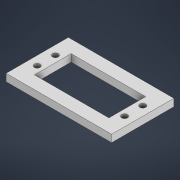
# Autodesk Inventor part: Servohalterung_v2
Saved by Autodesk Inventor 2021 (Build 250183000, 183)
## iProperties
Created: 2021-01-09
Part Number: Servohalterung_v2
Material: Generisch
Document SubType Name: Modeling
Designer: laure
Density: 1 g/cm^3
Appearance: Vorgabe
Author: laure
Autodesk Inventor part; units mm, degrees
ref_plane "YZ Plane" through (0, 0, 0) normal (1, 0, 0) x (0, 1, 0)
ref_plane "XZ Plane" through (0, 0, 0) normal (0, 1, 0) x (-1, 0, 0)
ref_plane "XY Plane" through (0, 0, 0) normal (0, 0, 1) x (1, 0, 0)
sketch "Skizze1" plane through (0, 0, 0) normal (0, 1, 0) x (-1, 0, 0)
  line L0 (20.5, -10.1) -> (-20.5, -10.1)
  line L1 (-20.5, -10.1) -> (-20.5, 10.1)
  line L2 (-20.5, 10.1) -> (20.5, 10.1)
  line L3 (20.5, 10.1) -> (20.5, -10.1)
  line L4 (0, -23.94) -> (0, 23.94) projected
  line L5 (-40.6, 0) -> (40.6, 0) projected
  line L6 (29, -17.1) -> (-29, -17.1)
  line L7 (-29, -17.1) -> (-29, 17.1)
  line L8 (-29, 17.1) -> (29, 17.1)
  line L9 (29, 17.1) -> (29, -17.1)
  point P0 (0, 0)
  dimension "d0" = 41
  dimension "d3" = 20.2
  dimension "d7" = 58
  dimension "d8" = 7
  constraints: 16 end point, 4 parallel, 2 horizontal, 2 perpendicular, 4 other
  measures "d0" distance between parallel lines of L1 L3
  measures "d3" distance of L2.end L0.start
  measures "d7" distance between parallel lines of L7 L9
  measures "d8" distance between parallel lines of L6 L0
extrude "Extrusion2" add sketch "Skizze1" along normal mid plane 4 contours L3 L5 L9 L6 L4 L0 | L4 L6 L7 L5 L1 L0 | L3 L2 L4 L8 L9 L5 | L5 L7 L8 L4 L2 L1
sketch "Skizze2" plane through (0, 2, 0) normal (0, 1, 0) x (1, 0, 0)
  circle A0 centre (-24, 5) radius 1.6
  circle A1 centre (-24, -5) radius 1.6
  line L0 (-29, 17.1) -> (-29, -17.1) projected
  line L1 (40.6, 0) -> (-40.6, 0) projected
  line L2 (0, 23.94) -> (0, -23.94) projected
  circle A2 centre (24, 5) radius 1.6
  circle A3 centre (24, -5) radius 1.6
  point P0 (0, 0)
  dimension "d11" = 3.2
  dimension "d12" = 3.2
  dimension "d13" = 5
  dimension "d14" = 5
  dimension "d15" = 10
  dimension "d16" = 5
  constraints: 4 centre point, 2 symmetric about line, 2 other
  measures "d11" diameter of A0
  measures "d12" diameter of A1
  measures "d13" distance from line of L0 A0.centre
  measures "d14" distance from line of L0 A1.centre
  measures "d15" distance of A1.centre A0.centre
  measures "d16" distance from line of L1 A0.centre
extrude "Extrusion3" cut sketch "Skizze2" against normal up to surface (4 mm away)
